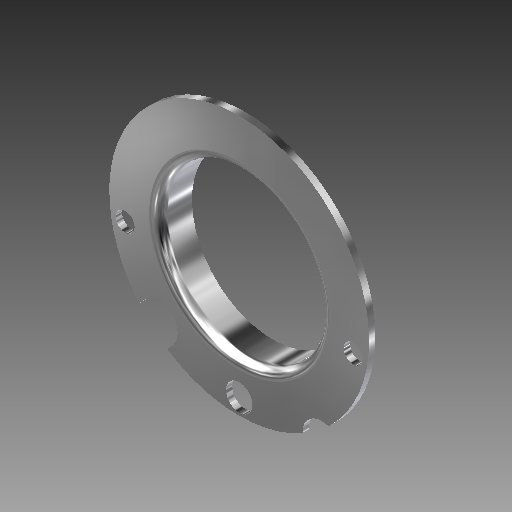
# Autodesk Inventor part: 403-02
Saved by Autodesk Inventor 2019 (Build 230136000, 136)
## iProperties
Company: Autodesk Inc.
Created: 2017-06-27
Part Number: 403-02
Material: Aluminum-6061
Document SubType Name: Modeling
Designer: Autodesk Inc.
Mass: 2.90581 g
Surface Area: 24.0141 cm^2
Volume: 1.07622 cm^3
Density: 2.7 g/cm^3
Appearance: Aluminum - Flat
Author: Inventor
Autodesk Inventor part; units mm, degrees
ref_plane "YZ Plane" through (0, 0, 0) normal (1, 0, 0) x (0, 1, 0)
ref_plane "XZ Plane" through (0, 0, 0) normal (0, 1, 0) x (-1, 0, 0)
ref_plane "XY Plane" through (0, 0, 0) normal (0, 0, 1) x (1, 0, 0)
sketch "Sketch1" plane through (0, 0, 0) normal (0, 0, 1) x (1, 0, 0)
  line L0 (0, 20.5) -> (1, 20.5)
  line L1 (1, 20.5) -> (1, 12.75)
  line L2 (1, 12.75) -> (0, 12.75)
  line L3 (0, 12.75) -> (0, 20.5)
  line L4 (1, 12.75) -> (5.3, 12.75)
  line L5 (5.3, 12.75) -> (5.3, 13.75)
  line L6 (5.3, 13.75) -> (1, 13.75)
  line L7 (1, 13.75) -> (1, 12.75)
  line L8 (0, 0) -> (7.1603, 0)
  dimension "d0" = 41
  dimension "d2" = 27.5
  dimension "d3" = 1
  dimension "d4" = 5.3
  constraints: 18 end point, 4 parallel, 4 perpendicular, 2 horizontal, 1 point on line
  measures "d0" diameter of L0 L8
  measures "d2" diameter of L6 L8
  measures "d3" distance of L4.end L5.end
  measures "d4" distance between parallel lines of L5 L3
revolve "Revolution1" add sketch "Sketch1" angle 360 about axis through (0, 0, 0) along (1, 0, 0)
fillet "Fillet1" radius 1.5 1 edges at (0, -12.75, 0)
fillet "Fillet1" radius 0.5 1 edges at (1, -13.75, 0)
sketch "Sketch2" plane through (0, 0, 0) normal (-1, 0, 0) x (0, 0, 1)
  line L0 (-18, -3) -> (18, -3) construction
  point P0 (0, 0)
  point P1 (0, -3)
  dimension "d8" = 36
  dimension "d9" = 3
  constraints: 2 end point, 1 horizontal, 1 midpoint, 1 vertical alignment
  measures "d8" distance of L0.start L0.end
  measures "d9" distance from line of point (0, 0) L0
hole "Hole1" at (0, -3, 18) at (0, -3, -18) direction (1, 0, 0) diameter 3 end through all
sketch "Sketch3" plane through (0, 0, 0) normal (-1, 0, 0) x (0, 0, 1)
  circle A0 centre (13, -17.7) radius 3
  circle A1 centre (-12.7, -14.1) radius 3
  line L0 (0, 0) -> (-12.7, -14.1) construction
  line L1 (-10.4709, -16.1078) -> (-11.3429, -17.0759)
  circle A2 centre (0, 0) radius 20.5 projected
  line L2 (-14.9291, -12.0922) -> (-15.8011, -13.0604)
  dimension "d17" = 13
  dimension "d18" = 17.7
  dimension "d19" = 12.7
  dimension "d20" = 14.1
  dimension "d21" = 6
  dimension "d22" = 6
  constraints: 6 end point, 4 point on circle, 2 centre point, 2 coincident, 2 parallel, 2 tangent
  measures "d17" horizontal distance of point (13, -17.7) L0.start
  measures "d18" vertical distance of L0.start point (13, -17.7)
  measures "d19" horizontal distance of L0.start point (-12.7, -14.1)
  measures "d20" vertical distance of L0.start point (-12.7, -14.1)
  measures "d21" diameter of A0
  measures "d22" diameter of A1
extrude "Extrusion1" cut sketch "Sketch3" against normal through all contours A0 A2 | A2 A0 | A2 A1 L1 | L2 A1 A2 | A1 A2 | A1 A2
sketch "Sketch4" plane through (0, 0, 0) normal (1, 0, 0) x (0, 1, 0)
  line L0 (0, 0) -> (-18, 0) construction
  dimension "d25" = 18
  constraints: 2 end point, 1 horizontal
  measures "d25" distance of L0.start L0.end
hole "Hole2" at (0, -18, 0) direction (1, 0, 0) diameter 4.2 end through all
body "Solid1"
